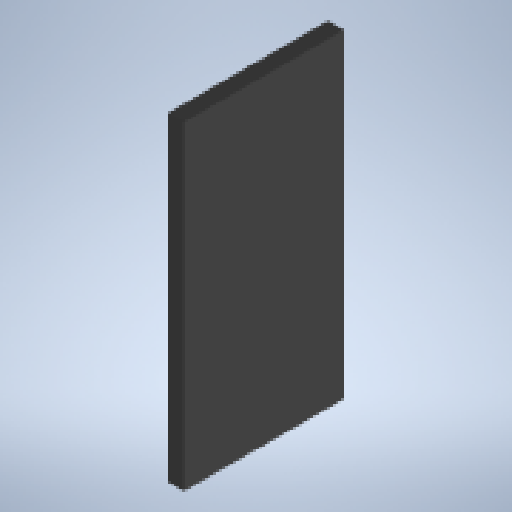
# Autodesk Inventor part: BremsbelagBreit
Saved by Autodesk Inventor 2025 (Build 290162010, 162A)
## iProperties
Created: 2025-01-23
Part Number: BremsbelagBreit
Material: Gummi
Document SubType Name: Modeling
Designer: Admin
Density: 0.93 g/cm^3
Appearance: Gummi - Schwarz
Author: Admin
Autodesk Inventor part; units mm, degrees
ref_plane "YZ Plane" through (0, 0, 0) normal (1, 0, 0) x (0, 1, 0)
ref_plane "XZ Plane" through (0, 0, 0) normal (0, 1, 0) x (-1, 0, 0)
ref_plane "XY Plane" through (0, 0, 0) normal (0, 0, 1) x (1, 0, 0)
sketch "Skizze1" plane through (0, 0, 0) normal (1, 0, 0) x (0, 1, 0)
  line L0 (0, 0) -> (-20, 0)
  line L1 (-20, 0) -> (-20, -40)
  line L2 (-20, -40) -> (0, -40)
  line L3 (0, -40) -> (0, 0)
  dimension "d0" = 20
  dimension "d1" = 40
  constraints: 8 end point, 2 parallel, 1 horizontal, 1 perpendicular
  measures "d0" distance of L2.end L1.end
  measures "d1" distance of L1.end L0.end
extrude "Extrusion1" add sketch "Skizze1" along normal blind 2
